Autodesk Fusion 360 part; units mm, degrees
note: some values were not read from the file. Set by a fixed rule: which sketch regions a step uses.
(part 3 of 3)
sketch "Sketch2" plane through (0, 0, 0) normal (0, 0, 1) x (1, 0, 0)
  line L0 (132.2365, -75.9165) -> (150.0405, -75.9165)
  line L1 (150.7462, -76.6369) -> (150.7462, -116.2783)
  line L2 (150.1207, -116.8682) -> (125.1075, -116.8682)
  line L3 (124.5583, -116.3407) -> (124.5583, -97.7967)
  line L4 (124.0741, -97.3063) -> (119.7549, -97.3063)
  line L5 (119.2267, -96.7788) -> (119.2267, -80.7164)
  arc A0 (150.7462, -76.6369) -> (150.0405, -75.9165) centre (150.0257, -76.6369) ccw
  arc A1 (150.1207, -116.8682) -> (150.7462, -116.2783) centre (150.1207, -116.2416) ccw
  arc A2 (124.5583, -116.3407) -> (125.1075, -116.8682) centre (125.1075, -116.3185) ccw
  arc A3 (124.5583, -97.7967) -> (124.0741, -97.3063) centre (124.0679, -97.7967) ccw
  arc A4 (119.2267, -96.7788) -> (119.7549, -97.3063) centre (119.7549, -96.778) ccw
  line L6 (132.2365, -75.9165) -> (119.2267, -75.9165)
  line L7 (119.2267, -75.9165) -> (119.2267, -80.7164)
  arc A5 (114.2267, -96.7766) -> (119.5583, -102.3028) centre (119.7549, -96.778) ccw
  line L8 (114.2267, -96.7766) -> (114.2267, -80.7164)
  line L9 (114.2267, -73.8739) -> (114.2267, -80.7164)
  line L10 (132.2365, -70.9165) -> (130.5504, -70.9165)
  line L11 (132.2365, -70.9165) -> (150.0674, -70.9165)
  arc A6 (155.7462, -76.6369) -> (150.0674, -70.9165) centre (150.0257, -76.6369) ccw
  line L12 (155.7462, -76.6369) -> (155.7462, -116.3517)
  arc A7 (150.1207, -121.8682) -> (155.7462, -116.3517) centre (150.1207, -116.2416) ccw
  line L13 (150.1207, -121.8682) -> (125.1075, -121.8682)
  arc A8 (119.5583, -116.3889) -> (125.1075, -121.8682) centre (125.1075, -116.3185) ccw
  line L14 (119.5583, -116.3889) -> (119.5583, -102.3028)
  line L15 (133.1519, -78.4856) -> (131.969, -76.4151)
  line L16 (131.969, -76.4151) -> (129.6822, -72.4126)
  line L17 (122.2117, -84.7318) -> (119.9639, -80.5591)
  line L18 (119.9639, -80.5591) -> (116.107, -73.3996)
  line L19 (124.0705, -97.7063) -> (119.7549, -97.7063)
  arc A9 (118.8267, -96.7774) -> (119.7549, -97.7063) centre (119.7549, -96.778) ccw
  line L20 (118.8267, -96.7774) -> (118.8267, -80.7164)
  line L21 (118.8267, -75.5165) -> (118.8267, -80.7164)
  line L22 (132.2365, -75.5165) -> (118.8267, -75.5165)
  line L23 (132.2365, -75.5165) -> (150.0442, -75.5165)
  arc A10 (151.1462, -76.6369) -> (150.0442, -75.5165) centre (150.0257, -76.6369) ccw
  line L24 (151.1462, -76.6369) -> (151.1462, -116.2886)
  arc A11 (150.1207, -117.2682) -> (151.1462, -116.2886) centre (150.1207, -116.2416) ccw
  line L25 (150.1207, -117.2682) -> (125.1075, -117.2682)
  arc A12 (124.1583, -116.3476) -> (125.1075, -117.2682) centre (125.1075, -116.3185) ccw
  line L26 (124.1583, -116.3476) -> (124.1583, -97.7967)
  arc A13 (124.1583, -97.7967) -> (124.0705, -97.7063) centre (124.0679, -97.7967) ccw
  arc A14 (130.5504, -70.9165) -> (129.6822, -72.4126) centre (130.5504, -71.9165) ccw
  arc A15 (116.107, -73.3996) -> (114.2267, -73.8739) centre (115.2267, -73.8739) ccw
  line L27 (133.0508, -78.8438) -> (122.4361, -84.7972)
  arc A16 (122.2117, -84.7318) -> (122.4361, -84.7972) centre (122.356, -84.6543) ccw
  arc A17 (133.0508, -78.8438) -> (133.1519, -78.4856) centre (132.9254, -78.615) ccw
  circle A18 centre (121.195, -95.3619) radius 1.1
  circle A19 centre (126.5232, -114.8824) radius 1.1
  circle A20 centre (148.6984, -114.9217) radius 1.1
  circle A21 centre (148.7631, -77.8933) radius 1.1
  point P0 (132.2365, -75.9165)
  point P1 (150.0405, -75.9165)
  point P2 (150.7462, -76.6369)
  point P3 (150.7462, -116.2783)
  point P4 (150.1207, -116.8682)
  point P5 (125.1075, -116.8682)
  point P6 (124.5583, -116.3407)
  point P7 (124.5583, -97.7967)
  point P8 (124.0741, -97.3063)
  point P9 (119.7549, -97.3063)
  point P10 (119.2267, -96.7788)
  point P11 (119.2267, -80.7164)
  point P12 (119.2267, -75.9165)
  point P13 (119.9639, -80.5591)
  point P14 (131.969, -76.4151)
  point P15 (122.2117, -84.7318)
  point P16 (119.9639, -80.5591)
  point P17 (133.1519, -78.4856)
  point P18 (133.0508, -78.8438)
  point P19 (122.4361, -84.7972)
  point P20 (121.195, -95.3619)
  point P21 (126.5232, -114.8824)
  point P22 (130.1874, -125.7456)
  point P23 (148.6984, -114.9217)
  point P24 (148.7631, -77.8933)
  dimension "d2" = 0.4
  dimension "d3" = 1
  dimension "d4" = 2.2
  dimension "d5" = 2.2
  dimension "d6" = 2.2
  dimension "d7" = 2.2
  constraint coincident P0 L0.start
  constraint coincident P1 L0.end
  constraint horizontal L0
  constraint coincident P2 L1.start
  constraint coincident P3 L1.end
  constraint perpendicular L0 L1
  constraint coincident P4 L2.start
  constraint coincident P5 L2.end
  constraint perpendicular L1 L2
  constraint coincident P6 L3.start
  constraint coincident P7 L3.end
  constraint perpendicular L0 L3
  constraint coincident P8 L4.start
  constraint coincident P9 L4.end
  constraint perpendicular L3 L4
  constraint coincident P10 L5.start
  constraint coincident P11 L5.end
  constraint perpendicular L4 L5
  constraint tangent L1 A0
  constraint tangent L2 A1
  constraint tangent L2 A2
  constraint tangent L3 A3
  constraint tangent L4 A4
  constraint coincident P12 L6.end
  constraint parallel L0 L6
  constraint perpendicular L6 L7
  constraint coincident P16 P13
  constraint coincident P17 L15.start
  constraint coincident P14 L15.end
  constraint parallel L15 L16
  constraint coincident P15 L17.start
  constraint parallel L17 L18
  constraint concentric A4 A5
  constraint parallel L5 L8
  constraint parallel L7 L9
  constraint parallel L6 L10
  constraint parallel L0 L11
  constraint concentric A0 A6
  constraint parallel L1 L12
  constraint concentric A1 A7
  constraint parallel L2 L13
  constraint concentric A2 A8
  constraint parallel L3 L14
  constraint tangent A7 L13
  constraint tangent A6 L12
  constraint tangent L13 A8
  constraint tangent L10 A14
  constraint tangent L16 A14
  constraint tangent L18 A15
  constraint tangent L9 A15
  constraint equal A14 A15
  constraint coincident P18 L27.start
  constraint coincident P19 L27.end
  constraint tangent L27 A16
  constraint tangent L15 A17
  constraint coincident P20 A18.centre
  constraint coincident P21 A19.centre
  constraint coincident P23 A20.centre
  constraint coincident P24 A21.centre
  measures "d3" radius of A14
  measures "d4" diameter of A18
  measures "d5" diameter of A19
  measures "d6" diameter of A20
  measures "d7" diameter of A21
extrude "Extrude1" add sketch "Sketch2" along normal blind 1 contours L0 L1 L2 L3 L4 L5 A0 A1 A2 A3 A4 L6 L7 L16 L18 L19 A9 L20 L21 L22 L23 A10 L24 A11 L25 A12 L26 A13 | L0 L1 L2 L3 L4 L5 A0 A1 A2 A3 A4 L6 L7 L15 L16 L17 L18 L27 A16 A17 makes body 1
extrude "Extrude2" add sketch "Sketch2" along normal blind 15 contours A5 L8 L9 L10 L11 A6 L12 A7 L13 A8 L14 L16 L18 L19 A9 L20 L21 L22 L23 A10 L24 A11 L25 A12 L26 A13 A14 A15 bodies 1
chamfer "Chamfer1" distance 1 angle 45 14 edges at (117.4669, -75.9238, 15) (114.9821, -72.9042, 15) (114.2267, -77.2951, 15) (114.2267, -88.7465, 15) (115.7764, -100.6164, 15) (119.5583, -109.3459, 15) (121.2083, -120.2675, 15) (137.6141, -121.8682, 15) (154.0602, -120.2589, 15) (155.7462, -96.4943, 15) (154.0854, -72.6067, 15) (140.3089, -70.9165, 15) (129.6855, -71.4146, 15) (130.5689, -73.9646, 15) on bodies 1
imported_body "Derived Base Feature1" makes body 2
move_body "Move1" bodies 2 to x (1, 0, 0) y (0, 1, 0) z (0, 0, 1) at (0, 0, 10)
scale "Scale1" factor 4 about (124.1583, -97.7967, 1) bodies 1
delete_body "RemoveBody1" bodies 2
scale "Scale2" factors (1, 1, 1.4) about (228.0077, -175.6824, 57) bodies 1
sketch "Sketch3" plane through (0, 0, -27) normal (0, 0, -1) x (1, 0, 0)
  circle A0 centre (222.3185, 166.2967) radius 4.4
  circle A1 centre (133.6177, 166.1395) radius 4.4
  circle A2 centre (112.3052, 88.0575) radius 4.4
  circle A3 centre (222.5773, 18.1831) radius 4.4
  line L0 (91.9532, 0.2081) -> (116.3718, 45.5369)
  arc A4 (117.2695, 45.7984) -> (116.3718, 45.5369) centre (116.949, 45.2269) ccw
  line L1 (117.2695, 45.7984) -> (159.7282, 21.9849)
  arc A5 (160.1327, 20.552) -> (159.7282, 21.9849) centre (159.2265, 21.0697) ccw
  line L2 (160.1327, 20.552) -> (146.2536, -3.7397)
  arc A6 (146.2536, -3.7397) -> (149.7267, -9.7241) centre (149.7267, -5.7241) ccw
  line L3 (149.7267, -9.7241) -> (227.7947, -9.7241)
  arc A7 (227.7947, -9.7241) -> (250.5099, 13.1573) centre (227.6279, 13.1573) ccw
  line L4 (250.5099, 13.1573) -> (250.5099, 172.0166)
  arc A8 (250.5099, 172.0166) -> (228.0077, 194.0824) centre (228.0077, 171.576) ccw
  line L5 (228.0077, 194.0824) -> (127.9551, 194.0824)
  arc A9 (127.9551, 194.0824) -> (105.7583, 172.1654) centre (127.9551, 171.8838) ccw
  line L6 (105.7583, 172.1654) -> (105.7583, 115.821)
  arc A10 (105.7583, 115.821) -> (84.4316, 93.716) centre (106.5447, 93.7218) ccw
  line L7 (84.4316, 93.716) -> (84.4316, 29.4755)
  line L8 (84.4316, 29.4755) -> (84.4316, 2.1052)
  arc A11 (84.4316, 2.1052) -> (91.9532, 0.2081) centre (88.4316, 2.1052) ccw
  line L9 (84.4316, 2.1052) -> (84.4316, -4.7241)
  line L10 (89.4316, -9.7241) -> (149.7267, -9.7241)
  arc A12 (84.4316, -4.7241) -> (89.4316, -9.7241) centre (89.4316, -4.7241) ccw
  circle A13 centre (112.625, 16.4) radius 1.6252
  arc A14 (250.516, 13.1573) -> (227.8009, -9.7241) centre (227.6341, 13.1573) cw
  line L11 (127.9613, 194.0824) -> (228.0139, 194.0824)
  line L12 (133.6239, 166.1395) -> (112.3114, 88.0575)
  arc A15 (228.0139, 194.0824) -> (250.516, 172.0166) centre (228.0139, 171.576) cw
  circle A16 centre (222.5835, 18.1831) radius 1.625
  arc A17 (84.4378, 93.716) -> (105.7645, 115.821) centre (106.5509, 93.7218) cw
  line L13 (112.625, 16.4) -> (222.5835, 18.1831)
  line L14 (222.3247, 166.2967) -> (133.6239, 166.1395)
  arc A18 (105.7645, 172.1654) -> (127.9613, 194.0824) centre (127.9613, 171.8838) cw
  arc A19 (89.4378, -9.7241) -> (84.4378, -4.7241) centre (89.4378, -4.7241) cw
  line L15 (250.516, 172.0166) -> (250.516, 13.1573)
  line L16 (222.5835, 18.1831) -> (222.3247, 166.2967)
  circle A20 centre (222.3247, 166.2967) radius 1.625
  circle A21 centre (133.6239, 166.1395) radius 1.625
  line L17 (84.4378, 29.4755) -> (84.4378, 93.716)
  line L18 (227.8009, -9.7241) -> (89.4378, -9.7241)
  circle A22 centre (112.3114, 88.0575) radius 1.625
  line L19 (112.3114, 88.0575) -> (112.625, 16.4)
  line L20 (105.7645, 115.821) -> (105.7645, 172.1654)
  line L21 (84.4378, -4.7241) -> (84.4378, 29.4755)
  point P0 (149.7267, -9.7241)
  point P1 (84.4316, 2.1052)
  point P2 (112.3052, 88.0575)
  point P3 (222.5773, 18.1831)
  point P4 (222.3185, 166.2967)
  point P5 (133.6177, 166.1395)
  dimension "d17" = 5
  constraint coincident P0 A6.end
  constraint coincident P1 L8.end
  constraint tangent A11 L9
  constraint tangent A6 L10
  constraint tangent L9 A12
  constraint tangent L10 A12
  constraint coincident P2 A2.centre
  constraint coincident P3 A3.centre
  constraint coincident P4 A0.centre
  constraint coincident P5 A1.centre
  measures "d17" radius of A12
extrude "Extrude3" add sketch "Sketch3" against normal blind 5.6 contours L0 A4 L1 A5 L2 A13 L13 L19 | L0 L2 A6 A11 L10 A13 L13 A19 L18 L19 L21 | A13 L13 L19 | A13 L13 L19 | A11 L9 A12 A19 L21 bodies 1
extrude "Extrude4" add sketch "Sketch3" against normal blind 5.6 contours A0 L14 L16 A20 | A0 L14 L16 A20 | A1 L12 L14 A21 | A1 L12 L14 A21 | A3 A16 L13 L16 | A3 A16 L13 L16 | A2 L12 A22 L19 | A2 L12 A22 L19 bodies 1
sketch "Sketch4" plane through (0, 0, 0) normal (0, 0, 1) x (-1, 0, 0)
  arc A0 (-125.871, 171.914) -> (-127.9015, 173.9515) centre (-128.65, 171.175) ccw
  line L0 (-127.9015, 173.9515) -> (-228.015, 173.9541)
  arc A1 (-228.015, 173.9541) -> (-230.3012, 171.6757) centre (-227.175, 170.825) ccw
  line L1 (-230.3012, 171.6757) -> (-230.375, 13.1141)
  arc A2 (-230.375, 13.1141) -> (-227.6585, 10.3811) centre (-226.65, 14.1) ccw
  line L2 (-227.6585, 10.3811) -> (-106.5581, 10.3259)
  arc A3 (-106.5581, 10.3259) -> (-104.5259, 12.3582) centre (-107.3, 13.1) ccw
  line L3 (-104.5259, 12.3582) -> (-104.535, 93.682)
  arc A4 (-104.535, 93.682) -> (-106.5668, 95.7147) centre (-107.3, 92.95) ccw
  line L4 (-106.5668, 95.7147) -> (-123.8363, 95.7243)
  arc A5 (-125.871, 97.7461) -> (-123.8363, 95.7243) centre (-123.1, 98.5) ccw
  line L5 (-125.871, 97.7461) -> (-125.871, 171.914)
  circle A6 centre (-222.325, 166.275) radius 1.625
  line L6 (-196.725, 150.9) -> (-196.725, 146.9)
  arc A7 (-197.725, 146.9) -> (-196.725, 146.9) centre (-197.225, 146.9) ccw
  line L7 (-197.725, 146.9) -> (-197.725, 150.9)
  arc A8 (-196.725, 150.9) -> (-197.725, 150.9) centre (-197.225, 150.9) ccw
  circle A9 centre (-205.175, 139.425) radius 6.1513
  circle A10 centre (-177.225, 138.9) radius 7
  line L8 (-196.675, 103.65) -> (-196.675, 99.65)
  arc A11 (-197.675, 99.65) -> (-196.675, 99.65) centre (-197.175, 99.65) ccw
  line L9 (-197.675, 99.65) -> (-197.675, 103.65)
  arc A12 (-196.675, 103.65) -> (-197.675, 103.65) centre (-197.175, 103.65) ccw
  line L10 (-186.225, 124.9) -> (-186.225, 122.9)
  arc A13 (-188.225, 122.9) -> (-186.225, 122.9) centre (-187.225, 122.9) ccw
  line L11 (-188.225, 122.9) -> (-188.225, 124.9)
  arc A14 (-186.225, 124.9) -> (-188.225, 124.9) centre (-187.225, 124.9) ccw
  circle A15 centre (-177.179, 91.6375) radius 7.9577
  circle A16 centre (-157.225, 148.9) radius 0.381
  circle A17 centre (-157.225, 143.9) radius 0.381
  circle A18 centre (-157.225, 133.9) radius 0.381
  circle A19 centre (-144.15, 139.425) radius 8.125
  circle A20 centre (-133.6, 166.125) radius 1.6258
  circle A21 centre (-157.225, 128.9) radius 0.381
  circle A22 centre (-157.175, 101.65) radius 0.381
  circle A23 centre (-157.175, 96.65) radius 0.381
  line L12 (-196.65, 56.6) -> (-196.65, 52.6)
  arc A24 (-197.65, 52.6) -> (-196.65, 52.6) centre (-197.15, 52.6) ccw
  line L13 (-197.65, 52.6) -> (-197.65, 56.6)
  arc A25 (-196.65, 56.6) -> (-197.65, 56.6) centre (-197.15, 56.6) ccw
  line L14 (-186.175, 77.65) -> (-186.175, 75.65)
  arc A26 (-188.175, 75.65) -> (-186.175, 75.65) centre (-187.175, 75.65) ccw
  line L15 (-188.175, 75.65) -> (-188.175, 77.65)
  arc A27 (-186.175, 77.65) -> (-188.175, 77.65) centre (-187.175, 77.65) ccw
  circle A28 centre (-205.075, 43.875) radius 6.1505
  circle A29 centre (-222.6, 18.175) radius 1.6502
  circle A30 centre (-177.15, 44.6) radius 7
  line L16 (-186.15, 30.6) -> (-186.15, 28.6)
  arc A31 (-188.15, 28.6) -> (-186.15, 28.6) centre (-187.15, 28.6) ccw
  line L17 (-188.15, 28.6) -> (-188.15, 30.6)
  arc A32 (-186.15, 30.6) -> (-188.15, 30.6) centre (-187.15, 30.6) ccw
  circle A33 centre (-157.175, 86.65) radius 0.381
  circle A34 centre (-157.175, 81.65) radius 0.381
  circle A35 centre (-157.15, 54.6) radius 0.381
  circle A36 centre (-124.14, 85.1) radius 0.5
  circle A37 centre (-132.125, 80.26) radius 0.5
  circle A38 centre (-132.125, 77.72) radius 0.5
  circle A39 centre (-132.125, 75.18) radius 0.5
  circle A40 centre (-132.125, 72.64) radius 0.5
  circle A41 centre (-128.072, 80.26) radius 0.508
  circle A42 centre (-127.818, 77.72) radius 0.508
  circle A43 centre (-128.072, 75.18) radius 0.508
  circle A44 centre (-127.818, 72.64) radius 0.508
  circle A45 centre (-124.135, 76.277) radius 0.508
  circle A46 centre (-121.6, 85.1) radius 0.5
  circle A47 centre (-119.06, 85.1) radius 0.5
  circle A48 centre (-116.52, 85.1) radius 0.5
  circle A49 centre (-112.275, 88.075) radius 1.6252
  circle A50 centre (-121.595, 76.023) radius 0.508
  circle A51 centre (-119.055, 76.277) radius 0.508
  circle A52 centre (-116.515, 76.023) radius 0.508
  circle A53 centre (-112.578, 80.26) radius 0.508
  circle A54 centre (-112.832, 77.72) radius 0.508
  circle A55 centre (-108.575, 80.25) radius 0.5
  circle A56 centre (-108.575, 77.71) radius 0.5
  circle A57 centre (-112.578, 75.18) radius 0.508
  circle A58 centre (-112.832, 72.64) radius 0.508
  circle A59 centre (-108.575, 75.17) radius 0.5
  circle A60 centre (-108.575, 72.63) radius 0.5
  circle A61 centre (-132.125, 70.1) radius 0.5
  circle A62 centre (-132.125, 67.56) radius 0.5
  circle A63 centre (-132.125, 65.02) radius 0.5
  circle A64 centre (-128.072, 70.1) radius 0.508
  circle A65 centre (-127.818, 67.56) radius 0.508
  circle A66 centre (-124.3, 70.11) radius 0.5
  circle A67 centre (-124.3, 67.57) radius 0.5
  circle A68 centre (-128.072, 65.02) radius 0.508
  circle A69 centre (-124.3, 65.03) radius 0.5
  circle A70 centre (-132.125, 62.48) radius 0.5
  circle A71 centre (-132.125, 59.94) radius 0.5
  circle A72 centre (-132.125, 57.4) radius 0.5
  circle A73 centre (-132.125, 54.86) radius 0.5
  circle A74 centre (-127.818, 62.48) radius 0.508
  circle A75 centre (-128.072, 59.94) radius 0.508
  circle A76 centre (-124.3, 62.49) radius 0.5
  circle A77 centre (-124.3, 59.95) radius 0.5
  circle A78 centre (-127.818, 57.4) radius 0.508
  circle A79 centre (-128.072, 54.86) radius 0.508
  circle A80 centre (-121.76, 70.11) radius 0.5
  circle A81 centre (-119.15, 70.11) radius 0.5
  circle A82 centre (-121.76, 67.57) radius 0.5
  circle A83 centre (-119.15, 67.57) radius 0.5
  circle A84 centre (-116.61, 70.11) radius 0.5
  circle A85 centre (-116.61, 67.57) radius 0.5
  circle A86 centre (-121.76, 65.03) radius 0.5
  circle A87 centre (-119.15, 65.03) radius 0.5
  circle A88 centre (-116.61, 65.03) radius 0.5
  circle A89 centre (-112.578, 70.1) radius 0.508
  circle A90 centre (-112.832, 67.56) radius 0.508
  circle A91 centre (-108.575, 70.09) radius 0.5
  circle A92 centre (-108.575, 67.55) radius 0.5
  circle A93 centre (-112.578, 65.02) radius 0.508
  circle A94 centre (-108.575, 65.01) radius 0.5
  circle A95 centre (-121.76, 62.49) radius 0.5
  circle A96 centre (-119.15, 62.49) radius 0.5
  circle A97 centre (-121.76, 59.95) radius 0.5
  circle A98 centre (-119.15, 59.95) radius 0.5
  circle A99 centre (-116.61, 62.49) radius 0.5
  circle A100 centre (-116.61, 59.95) radius 0.5
  circle A101 centre (-112.832, 62.48) radius 0.508
  circle A102 centre (-112.578, 59.94) radius 0.508
  circle A103 centre (-108.575, 62.47) radius 0.5
  circle A104 centre (-108.575, 59.93) radius 0.5
  circle A105 centre (-112.832, 57.4) radius 0.508
  circle A106 centre (-112.578, 54.86) radius 0.508
  circle A107 centre (-108.575, 57.39) radius 0.5
  circle A108 centre (-108.575, 54.85) radius 0.5
  circle A109 centre (-157.15, 49.6) radius 0.381
  circle A110 centre (-157.15, 39.6) radius 0.381
  circle A111 centre (-157.15, 34.6) radius 0.381
  circle A112 centre (-144.2, 43.9) radius 8.125
  circle A113 centre (-132.125, 52.32) radius 0.5
  circle A114 centre (-132.125, 49.78) radius 0.5
  circle A115 centre (-132.125, 47.24) radius 0.5
  circle A116 centre (-132.125, 44.7) radius 0.5
  circle A117 centre (-127.818, 52.32) radius 0.508
  circle A118 centre (-128.072, 49.78) radius 0.508
  circle A119 centre (-127.818, 47.24) radius 0.508
  circle A120 centre (-128.072, 44.7) radius 0.508
  circle A121 centre (-132.125, 42.16) radius 0.5
  circle A122 centre (-132.125, 39.62) radius 0.5
  circle A123 centre (-132.125, 37.08) radius 0.5
  circle A124 centre (-132.125, 34.54) radius 0.5
  circle A125 centre (-127.818, 42.16) radius 0.508
  circle A126 centre (-128.072, 39.62) radius 0.508
  circle A127 centre (-127.818, 37.08) radius 0.508
  circle A128 centre (-128.072, 34.54) radius 0.508
  circle A129 centre (-112.832, 52.32) radius 0.508
  circle A130 centre (-112.578, 49.78) radius 0.508
  circle A131 centre (-108.575, 52.31) radius 0.5
  circle A132 centre (-108.575, 49.77) radius 0.5
  circle A133 centre (-112.832, 47.24) radius 0.508
  circle A134 centre (-112.578, 44.7) radius 0.508
  circle A135 centre (-108.575, 47.23) radius 0.5
  circle A136 centre (-108.575, 44.69) radius 0.5
  circle A137 centre (-112.832, 42.16) radius 0.508
  circle A138 centre (-112.578, 39.62) radius 0.508
  circle A139 centre (-108.575, 42.15) radius 0.5
  circle A140 centre (-108.575, 39.61) radius 0.5
  circle A141 centre (-112.832, 37.08) radius 0.508
  circle A142 centre (-112.578, 34.54) radius 0.508
  circle A143 centre (-108.575, 37.07) radius 0.5
  circle A144 centre (-108.575, 34.53) radius 0.5
  circle A145 centre (-132.125, 32) radius 0.5
  circle A146 centre (-127.818, 32) radius 0.508
  circle A147 centre (-112.832, 32) radius 0.508
  circle A148 centre (-108.575, 31.99) radius 0.5
  circle A149 centre (-112.275, 16.4) radius 1.6252
  circle A150 centre (-112.275, 16.4) radius 1.6252
  constraint concentric A149 A150
extrude "Extrude6" cut sketch "Sketch4" against normal blind 55 contours A149 A150 bodies 1
named bodies: "Body1 (1)"
